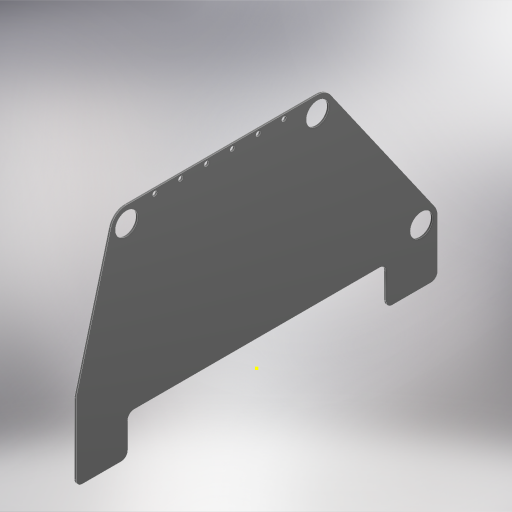
# Autodesk Inventor part: side 1.1
Saved by Autodesk Inventor 2023 (Build 270158000, 158)
## iProperties
Created: 2023-07-16
Part Number: side 1.1
Material: Acetal Resin, Black
Document SubType Name: Modeling
Designer: aaron
Density: 1.425 g/cm^3
Appearance: Smooth - Black
Author: aaron
Autodesk Inventor part; units mm, degrees
ref_plane "YZ Plane" through (0, 0, 0) normal (1, 0, 0) x (0, 1, 0)
ref_plane "XZ Plane" through (0, 0, 0) normal (0, 1, 0) x (-1, 0, 0)
ref_plane "XY Plane" through (0, 0, 0) normal (0, 0, 1) x (1, 0, 0)
sketch "Sketch1" plane through (0, 0, 0) normal (1, 0, 0) x (0, 1, 0)
  line L0 (-12.7, -177.8) -> (12.7, -177.8)
  line L1 (12.7, -177.8) -> (12.7, 177.8)
  line L2 (12.7, 177.8) -> (-12.7, 177.8)
  line L3 (-12.7, 177.8) -> (-12.7, -177.8)
  line L4 (-12.7, -177.8) -> (12.7, 177.8) construction
  line L5 (12.7, -177.8) -> (-12.7, 177.8) construction
  line L6 (12.7, -101.6) -> (12.7, 177.8)
  line L7 (12.7, 177.8) -> (25.4, 177.8)
  line L8 (25.4, 177.8) -> (25.4, -177.8)
  line L9 (25.4, -177.8) -> (12.7, -177.8)
  line L10 (12.7, -177.8) -> (12.7, 177.8)
  line L11 (25.4, 177.8) -> (203.2, 177.8)
  line L12 (203.2, 177.8) -> (203.2, -177.8)
  line L13 (203.2, -177.8) -> (25.4, -177.8)
  line L14 (25.4, -177.8) -> (25.4, 177.8)
  circle A0 centre (41.275, -161.925) radius 15.875
  circle A1 centre (187.325, -59.6597) radius 15.875
  line L15 (41.275, -161.925) -> (203.2, -48.5439)
  line L16 (41.275, -161.925) -> (238.9489, -161.925) construction
  line L17 (196.4305, -72.6637) -> (50.3805, -174.929)
  circle A2 centre (187.325, -59.6597) radius 10.9537
  circle A3 centre (41.275, -161.925) radius 10.9538
  point P0 (0, 0)
  point P1 (203.2, -59.6597)
  point P2 (41.275, -177.8)
  dimension "d7" = 31.75
  dimension "d8" = 31.75
  dimension "d0" = 25.4
  dimension "d1" = 355.6
  dimension "d4" = 12.7
  dimension "d5" = 177.8
  dimension "d6" = 355.6
  dimension "d9" = 35
  dimension "d10" = 21.9075
  dimension "d11" = 21.9075
  constraints: 36 end point, 7 parallel, 5 horizontal, 3 perpendicular, 2 centre point, 2 coincident, 2 midpoint, 2 point on line, 2 vertical, 1 equal length, 7 other
  measures "d0" distance of L2.end L1.end
  measures "d1" distance of L1.end L0.end
  measures "d4" distance of L8.end L9.end
  measures "d5" distance of L12.end L13.end
  measures "d6" distance of L11.end L12.end
  measures "d9" angle of L16 L15
  measures "d10" diameter of A2
  measures "d11" diameter of A3
extrude "Extrusion1" add sketch "Sketch1" along normal blind 1.5875 contours L3 L2 L1 L0 | L1 L7 L8 L9 | L8 A0 L13 | L8 L11 L12 L15 A1 A0 | A0 | L15 A1 L17 A0 | L15 A2 A1 | A1 L15 A2 | A1 L15 L12
sketch "Sketch2" plane through (1.5875, 0, 0) normal (1, 0, 0) x (0, 0, -1)
  line L0 (-177.8, -12.7) -> (177.8, -12.7) projected
  line L1 (-127, -12.7) -> (127, -12.7)
  line L2 (127, -12.7) -> (127, 25.4)
  line L3 (127, 25.4) -> (-127, 25.4)
  line L4 (-127, 25.4) -> (-127, -12.7)
  line L5 (-177.8, 203.2) -> (-177.8, -12.7) projected
  line L6 (177.8, -12.7) -> (177.8, 41.275) projected
  point P0 (0, 0)
  point P1 (127, -12.7)
  dimension "d14" = 38.1
  dimension "d15" = 50.8
  dimension "d16" = 50.8
  constraints: 8 end point, 2 parallel, 1 horizontal, 1 perpendicular, 1 point on line
  measures "d14" distance between parallel lines of L0 L3
  measures "d15" distance between parallel lines of L5 L4
  measures "d16" distance between parallel lines of L6 L2
extrude "Extrusion2" cut sketch "Sketch2" against normal blind 1.5875
sketch "Sketch3" plane through (1.5875, 0, 0) normal (1, 0, 0) x (0, 0, -1)
  line L0 (-177.8, 203.2) -> (-177.8, -12.7) projected
  line L1 (-177.8, -12.7) -> (-177.8, 63.5)
  line L2 (-177.8, 63.5) -> (-140.3675, 203.2)
  line L3 (59.6597, 203.2) -> (-177.8, 203.2) projected
  circle A0 centre (-128.1862, 187.325) radius 15.875
  circle A1 centre (-128.1862, 187.325) radius 10.9537
  point P0 (0, 0)
  point P1 (-143.5203, 191.4338)
  point P2 (-128.1862, 203.2)
  dimension "d19" = 76.2
  dimension "d20" = 165
  dimension "d23" = 31.75
  dimension "d24" = 21.9075
  constraints: 4 end point, 2 centre point, 2 point on line, 2 tangent, 1 coincident
  measures "d19" distance of L0.end L1.end
  measures "d20" angle of L1 L2
  measures "d23" diameter of A0
  measures "d24" diameter of A1
extrude "Extrusion3" cut sketch "Sketch3" against normal blind 1.5875 contours L3 L2 L0 | L3 A0 L2 | A1
fillet "Fillet1" radius 6.35 6 edges at (0.7937, -12.7, 127) (0.7937, -12.7, 177.8) (0.7937, 25.4, 127) (0.7937, 25.4, -127) (0.7937, -12.7, -127) (0.7937, -12.7, -177.8)
sketch "Sketch4" plane through (1.5875, 0, 0) normal (1, 0, 0) x (0, 0, -1)
  point P0 (0, 0)
sketch "Sketch5" plane through (1.5875, 0, 0) normal (1, 0, 0) x (0, 0, -1)
  circle A0 centre (59.6597, 187.325) radius 10.9537 projected
  circle A1 centre (59.6597, 187.325) radius 25.4
  circle A2 centre (161.925, 41.275) radius 10.9538 projected
  circle A3 centre (161.925, 41.275) radius 25.4
  circle A4 centre (26.7321, 198.9667) radius 9.525
  circle A5 centre (26.7321, 198.9667) radius 4.2333
  line L0 (59.6597, 203.2) -> (-128.1862, 203.2) projected
  circle A6 centre (26.7321, 198.9667) radius 2.159
  point P0 (0, 0)
  dimension "d26" = 50.8
  dimension "d27" = 50.8
  dimension "d28" = 19.05
  dimension "d29" = 8.4667
  dimension "d30" = 4.318
  constraints: 5 centre point, 4 coincident, 2 tangent
  measures "d26" diameter of A1
  measures "d27" diameter of A3
  measures "d28" diameter of A4
  measures "d29" diameter of A5
  measures "d30" diameter of A6
extrude "Extrusion4" cut sketch "Sketch5" against normal blind 1.5875 contours A6
pattern_linear "Rectangular Pattern1" count 6 spacing 25.4 along (0, 0, 1) of "Extrusion4"
body "Solid1"
